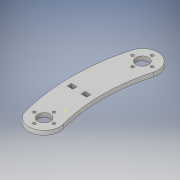
# Autodesk Inventor part: fem
Saved by Autodesk Inventor 2019 (Build 230136000, 136)
## iProperties
Created: 2023-04-15
Part Number: fem
Material: Generic
Document SubType Name: Modeling
Designer: Analuam
Density: 1 g/cm^3
Appearance: Default
Author: Analuam
Autodesk Inventor part; units mm, degrees
ref_plane "YZ Plane" through (0, 0, 0) normal (1, 0, 0) x (0, 1, 0)
ref_plane "XZ Plane" through (0, 0, 0) normal (0, 1, 0) x (-1, 0, 0)
ref_plane "XY Plane" through (0, 0, 0) normal (0, 0, 1) x (1, 0, 0)
sketch "Sketch1" plane through (0, 0, 0) normal (0, 1, 0) x (-1, 0, 0)
  arc A0 (13.7652, 13.7563) -> (-7.6488, 8.7996) centre (2.9529, 11.7331) ccw
  arc A1 (-7.6488, -55.3335) -> (13.7652, -60.2902) centre (2.9529, -58.2669) ccw
  arc A2 (-7.6723, -55.4199) -> (-7.6723, 8.8861) centre (-125.5725, -23.2669) ccw
  circle A3 centre (2.9529, 11.7331) radius 4.5
  circle A4 centre (2.9529, -58.2669) radius 4.5
  circle A5 centre (2.9529, 4.7331) radius 1
  circle A6 centre (9.9529, 11.7331) radius 1
  circle A7 centre (2.9529, 18.7331) radius 1
  circle A8 centre (-4.0471, 11.7331) radius 1
  circle A9 centre (2.9529, -65.2669) radius 1
  circle A10 centre (9.9529, -58.2669) radius 1
  circle A11 centre (2.9529, -51.2669) radius 1
  circle A12 centre (-4.0471, -58.2669) radius 1
  line L0 (14.3609, -16.1054) -> (10.3609, -16.1054)
  line L1 (10.3609, -16.1054) -> (10.3609, -19.1054)
  line L2 (10.3609, -19.1054) -> (14.3609, -19.1054)
  line L3 (14.3609, -19.1054) -> (14.3609, -16.1054)
  line L4 (14.3609, -11.7669) -> (10.3609, -14.7669) construction
  line L5 (10.3609, -11.7669) -> (14.3609, -14.7669) construction
  line L6 (0.5448, -16.1054) -> (4.5448, -16.1054)
  line L7 (4.5448, -16.1054) -> (4.5448, -19.1054)
  line L8 (4.5448, -19.1054) -> (0.5448, -19.1054)
  line L9 (0.5448, -19.1054) -> (0.5448, -16.1054)
  arc A13 (13.7652, -60.2902) -> (13.7652, 13.7563) centre (-124.6252, -23.2669) ccw
  line L10 (12.3609, -13.2669) -> (12.3609, -13.2669)
  line L11 (10.3609, -18.6054) -> (4.5448, -18.6054)
  line L12 (7.4529, -18.6054) -> (7.4529, -17.6054)
  point P0 (0, 0)
  dimension "d0" = 22
  dimension "d1" = 22
  dimension "d2" = 70
  dimension "d3" = 9
  dimension "d4" = 9
  dimension "d6" = 2
  dimension "d9" = 360
  dimension "d13" = 2
  dimension "d16" = 360
  dimension "d21" = 4
  dimension "d22" = 3
  dimension "d26" = 5.8161
  dimension "d27" = 13.8161
  dimension "d28" = 0
  dimension "d30" = 1
  constraints: 26 end point, 14 centre point, 12 point on circle, 2 coincident, 2 parallel, 2 vertical, 1 horizontal, 1 midpoint, 1 perpendicular, 18 other
  measures "d0" diameter of A0
  measures "d1" diameter of A1
  measures "d2" distance of A1.centre A0.centre
  measures "d3" diameter of A3
  measures "d4" diameter of A4
  measures "d6" diameter of A5
  measures "d13" diameter of A9
  measures "d21" distance of L2.end L1.end
  measures "d22" distance of L1.end L0.end
  measures "d26" distance between parallel lines of L7 L1
  measures "d27" distance between parallel lines of L9 L3
  measures "d28" distance of L10.start L10.end
  measures "d30" distance of L12.start L12.end
extrude "Extrusion1" add sketch "Sketch1" along normal blind 3
sketch "Sketch2" plane through (0, 3, 0) normal (0, 1, 0) x (1, 0, 0)
  point P0 (0, 0)
sketch "Sketch3" plane through (0, 3, 0) normal (0, 1, 0) x (1, 0, 0)
  point P0 (0, 0)
body "Solid1"
